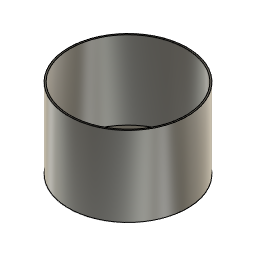
S(min)-all v4 (Autodesk Fusion 360 design; units mm, degrees)
Autodesk Fusion 360 part; units mm, degrees
sketch "スケッチ1" plane through (0, 0, 0) normal (0, 0, 1) x (1, 0, 0)
  circle A0 centre (0, 0) radius 39.9295
  circle A1 centre (0, 0) radius 40.9295
  dimension "d1" = 79.8589
  dimension "d2" = 81.8589
  constraint coincident A0.centre A1.centre
  measures "d1" diameter of A0
  measures "d2" diameter of A1
extrude "押し出し1" add sketch "スケッチ1" along normal blind 1 contours A0
extrude "押し出し2" add sketch "スケッチ1" along normal blind 55
equation "d1 = ( 39.929454246127 * 2 ) * 1 mm"
equation "d2 = d1 + 2 mm"
